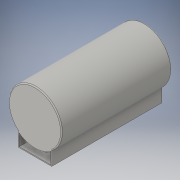
# Autodesk Inventor part: Tank
Saved by Autodesk Inventor 2016 (Build 200138000, 138)
## iProperties
Created: 2018-07-07
Part Number: Tank
Material: Generic
Document SubType Name: Modeling
Designer: Kade
Density: 1 g/cm^3
Appearance: Default
Author: Kade
Autodesk Inventor part; units mm, degrees
ref_plane "YZ Plane" through (0, 0, 0) normal (1, 0, 0) x (0, 1, 0)
ref_plane "XZ Plane" through (0, 0, 0) normal (0, 1, 0) x (-1, 0, 0)
ref_plane "XY Plane" through (0, 0, 0) normal (0, 0, 1) x (1, 0, 0)
sketch "Sketch6" plane through (0, 0, 0) normal (0, 0, 1) x (1, 0, 0)
  circle A0 centre (0, 0) radius 88.9
  dimension "d25" = 177.8
  constraints: 1 centre point, 1 coincident
  measures "d25" diameter of A0
extrude "Extrusion6" add sketch "Sketch6" along normal blind 368.3
sketch "Sketch7" plane through (0, 0, 368.3) normal (0, 0, 1) x (1, 0, 0)
  circle A0 centre (0, 0) radius 88.9 projected
  line L0 (55.8771, -69.1444) -> (55.8771, -114.3)
  line L1 (-55.8771, -69.1444) -> (-55.8771, -114.3)
  line L2 (-55.8771, -114.3) -> (55.8771, -114.3)
  arc A1 (-55.8771, -69.1444) -> (55.8771, -69.1444) centre (0, 0) ccw
  line L3 (52.7021, -111.125) -> (52.7021, -75.5003)
  arc A2 (-52.7021, -75.5003) -> (52.7021, -75.5003) centre (0, 0) ccw
  line L4 (-52.7021, -75.5003) -> (-52.7021, -111.125)
  line L5 (-52.7021, -111.125) -> (52.7021, -111.125)
  dimension "d29" = 3.175
  constraints: 12 end point, 6 point on circle, 2 centre point, 2 perpendicular, 2 vertical, 1 concentric, 3 other
  measures "d29" distance between parallel lines of L2 L5
extrude "Extrusion7" add sketch "Sketch7" against normal blind 368.3 contours A0 L0 L2 L1
fillet "Fillet1" radius 3.175 4 edges at (0, 88.9, 368.3) (0, 88.9, 0) (0, -92.075, 368.3) (0, -92.075, 0)
body "Solid2"
